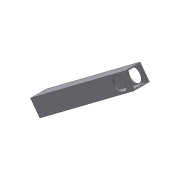
# Autodesk Inventor part: Shovel_RollerMount
Saved by Autodesk Inventor 2012 (Build 160160000, 160)
## iProperties
Created: 2013-01-29
Part Number: Shovel_RollerMount
Material: Aluminum-6061
Document SubType Name: Modeling
Designer: JesseK
Density: 2.71 g/cm^3
Mass: 74.7246 g
Surface Area: 352.626 cm^2
Volume: 27.5737 cm^3
Author: JesseK
Autodesk Inventor part; units mm, degrees
ref_plane "YZ Plane" through (0, 0, 0) normal (1, 0, 0) x (0, 1, 0)
ref_plane "XZ Plane" through (0, 0, 0) normal (0, 1, 0) x (-1, 0, 0)
ref_plane "XY Plane" through (0, 0, 0) normal (0, 0, 1) x (1, 0, 0)
sketch "Sketch1" plane through (0, 0, 0) normal (0, 0, 1) x (1, 0, 0)
  line L0 (-42.6455, -61.8334) -> (-57.8855, -41.5134)
  line L1 (-57.8855, -41.5134) -> (94.5145, 72.7866)
  line L2 (94.5145, 72.7866) -> (109.7545, 52.4666)
  line L3 (109.7545, 52.4666) -> (-42.6455, -61.8334)
  point P0 (0, 0)
  dimension "d0" = 25.4
  dimension "d1" = 190.5
  constraints: 8 end point, 2 parallel, 1 perpendicular
  measures "d0" distance of L1.end L2.end
  measures "d1" distance of L2.end L0.start
extrude "Extrusion1" add sketch "Sketch1" along normal blind 25.4
shell "Shell1" thickness 1.5875 removed faces 2 at (-47.7255, -55.0601, 8.4667) at (99.5945, 66.0133, 16.9333)
sketch "Sketch2" plane through (0, 0, 25.4) normal (0, 0, 1) x (1, 0, 0)
  line L0 (109.7545, 52.4666) -> (-42.6455, -61.8334) projected
  line L1 (94.5145, 72.7866) -> (109.7545, 52.4666) projected
  circle A0 centre (86.8945, 51.1966) radius 11.1125
  point P0 (0, 0)
  dimension "d5" = 22.225
  dimension "d6" = 12.7
  dimension "d7" = 19.05
  constraints: 1 centre point
  measures "d5" diameter of A0
  measures "d6" distance from line of L0 A0.centre
  measures "d7" distance from line of L1 A0.centre
extrude "Extrusion2" cut sketch "Sketch2" against normal through all
body "Solid1"
